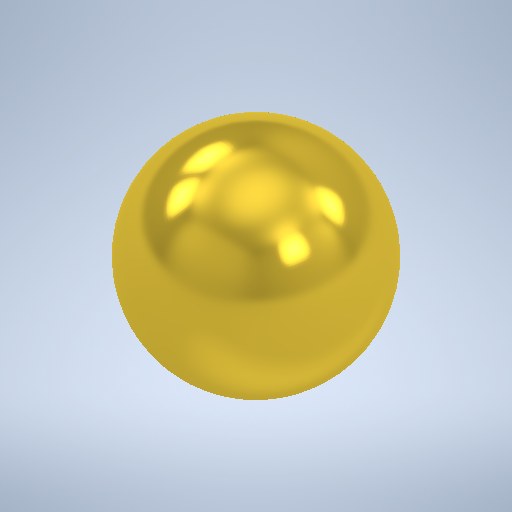
# Autodesk Inventor part: Ball
Saved by Autodesk Inventor 2025.1 (Build 291241000, 241)
## iProperties
Created: 2024-08-09
Part Number: Ball
Material: Generic
Document SubType Name: Modeling
Designer: vedan
Density: 1 g/cm^3
Appearance: Metal 2400F Hot
Author: vedan
Autodesk Inventor part; units mm, degrees
ref_plane "YZ Plane" through (0, 0, 0) normal (1, 0, 0) x (0, 1, 0)
ref_plane "XZ Plane" through (0, 0, 0) normal (0, 1, 0) x (-1, 0, 0)
ref_plane "XY Plane" through (0, 0, 0) normal (0, 0, 1) x (1, 0, 0)
sketch "Sketch1" plane through (0, 0, 0) normal (0, 0, 1) x (1, 0, 0)
  arc A0 (0, -12) -> (0, 12) centre (0, 0) ccw
  line L0 (0, 12) -> (0, -12) construction
  line L1 (0, 12) -> (0, -12)
  point P0 (12, 0)
  dimension "d1" = 12
  constraints: 4 end point, 4 point on circle, 1 centre point, 1 coincident, 1 collinear, 1 midpoint
  measures "d1" distance of point (12, 0) point (0, 0)
revolve "Revolution1" add sketch "Sketch1" angle 360 about axis through (0, 12, 0) along (0, -1, 0)
body "Solid1"
